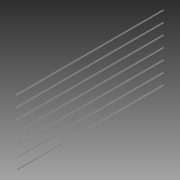
# Autodesk Inventor part: Left Cable
Saved by Autodesk Inventor 2015 (Build 190159000, 159)
## iProperties
Created: 2014-05-30
Part Number: Left Cable
Material: Steel, Wrought
Document SubType Name: Modeling
Designer: Haden
Density: 7.85 g/cm^3
Appearance: Steel
Author: Haden
Autodesk Inventor part; units mm, degrees
ref_plane "YZ Plane" through (0, 0, 0) normal (1, 0, 0) x (0, 1, 0)
ref_plane "XZ Plane" through (0, 0, 0) normal (0, 1, 0) x (-1, 0, 0)
ref_plane "XY Plane" through (0, 0, 0) normal (0, 0, 1) x (1, 0, 0)
sketch "Sketch1" plane through (0, 0, 0) normal (0, 0, 1) x (1, 0, 0)
  circle A0 centre (0, 0) radius 4.7625
  circle A1 centre (0, 101.6) radius 4.7625
  circle A2 centre (0, 203.2) radius 4.7625
  circle A3 centre (0, 304.8) radius 4.7625
  circle A4 centre (0, 406.4) radius 4.7625
  circle A5 centre (0, 508) radius 4.7625
  circle A6 centre (0, 609.6) radius 4.7625
  dimension "d0" = 9.525
  dimension "d3" = 101.6
  dimension "d4" = 101.6
  dimension "d5" = 101.6
  dimension "d6" = 101.6
  dimension "d7" = 101.6
  dimension "d10" = 101.6
  constraints: 7 centre point, 6 equal radius, 6 vertical alignment, 1 coincident
  measures "d0" diameter of A0
  measures "d3" distance of A1.centre point (0, 0)
  measures "d4" distance of A2.centre A1.centre
  measures "d5" distance of A3.centre A2.centre
  measures "d6" distance of A4.centre A3.centre
  measures "d7" distance of A5.centre A4.centre
  measures "d10" distance of A6.centre A5.centre
extrude "Extrusion2" add sketch "Sketch1" along normal blind 1377.188
body "Solid2"
